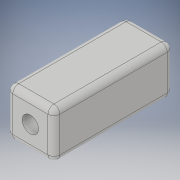
# Autodesk Inventor part: Square-Circle-Adapter V1D1
Saved by Autodesk Inventor 2017 (Build 210142000, 142)
## iProperties
Created: 2017-12-22
Part Number: Square-Circle-Adapter V1D1
Material: Generic
Document SubType Name: Modeling
Designer: Tripl_000
Density: 1 g/cm^3
Appearance: Default
Author: Tripl_000
Autodesk Inventor part; units mm, degrees
ref_plane "YZ Plane" through (0, 0, 0) normal (1, 0, 0) x (0, 1, 0)
ref_plane "XZ Plane" through (0, 0, 0) normal (0, 1, 0) x (-1, 0, 0)
ref_plane "XY Plane" through (0, 0, 0) normal (0, 0, 1) x (1, 0, 0)
sketch "Sketch1" plane through (0, 0, 0) normal (0, 0, 1) x (1, 0, 0)
  line L0 (-7.9, 7.9) -> (7.9, 7.9)
  line L1 (7.9, 7.9) -> (7.9, -7.9)
  line L2 (7.9, -7.9) -> (-7.9, -7.9)
  line L3 (-7.9, -7.9) -> (-7.9, 7.9)
  line L4 (-7.9, 7.9) -> (7.9, -7.9) construction
  line L5 (7.9, 7.9) -> (-7.9, -7.9) construction
  point P0 (0, 0)
  dimension "d0" = 15.8
  dimension "d1" = 15.8
  constraints: 12 end point, 2 midpoint, 2 parallel, 1 horizontal, 1 perpendicular
  measures "d0" distance of L2.end L0.start
  measures "d1" distance of L0.start L0.end
extrude "Extrusion1" add sketch "Sketch1" along normal blind 15
sketch "Sketch2" plane through (0, 0, 15) normal (0, 0, 1) x (1, 0, 0)
  line L0 (-6.4, 6.4) -> (6.4, 6.4)
  line L1 (6.4, 6.4) -> (6.4, -6.4)
  line L2 (6.4, -6.4) -> (-6.4, -6.4)
  line L3 (-6.4, -6.4) -> (-6.4, 6.4)
  line L4 (-6.4, 6.4) -> (6.4, -6.4) construction
  line L5 (6.4, 6.4) -> (-6.4, -6.4) construction
  point P0 (0, 0)
  dimension "d4" = 12.8
  dimension "d5" = 12.8
  constraints: 12 end point, 2 midpoint, 2 parallel, 1 horizontal, 1 perpendicular
  measures "d4" distance of L0.end L1.end
  measures "d5" distance of L0.start L0.end
extrude "Extrusion2" cut sketch "Sketch2" against normal through all
sketch "Sketch3" plane through (0, 0, 15) normal (0, 0, 1) x (1, 0, 0)
  line L0 (7.9, -7.9) -> (-7.9, -7.9) projected
  line L1 (-7.9, 7.9) -> (7.9, 7.9)
  line L2 (7.9, 7.9) -> (7.9, -7.9)
  line L3 (7.9, -7.9) -> (-7.9, -7.9)
  line L4 (-7.9, -7.9) -> (-7.9, 7.9)
  point P0 (0, 0)
  constraints: 8 end point, 2 parallel, 1 horizontal, 1 perpendicular
extrude "Extrusion3" add sketch "Sketch3" along normal blind 25
sketch "Sketch4" plane through (0, 0, 40) normal (0, 0, 1) x (1, 0, 0)
  circle A0 centre (0, 0) radius 2.75
  dimension "d10" = 5.5
  constraints: 1 centre point, 1 coincident
  measures "d10" diameter of A0
extrude "Extrusion4" cut sketch "Sketch4" against normal through all
fillet "Fillet1" radius 2 4 edges at (-6.4, 6.4, 7.5) (6.4, 6.4, 7.5) (6.4, -6.4, 7.5) (-6.4, -6.4, 7.5)
fillet "Fillet2" radius 2 8 edges at (5.8142, 5.8142, 15) (6.4, 0, 15) (5.8142, -5.8142, 15) (0, -6.4, 15) (-5.8142, -5.8142, 15) (-6.4, 0, 15) (-5.8142, 5.8142, 15) (0, 6.4, 15)
fillet "Fillet3" radius 2 12 edges at (-7.9, 7.9, 20) (7.9, 7.9, 20) (-7.9, -7.9, 20) (7.9, -7.9, 20) (7.9, 0, 0) (0, -7.9, 0) (-7.9, 0, 0) (0, 7.9, 0) (0, 7.9, 40) (-7.9, 0, 40) (7.9, 0, 40) (0, -7.9, 40)
body "Solid1"
